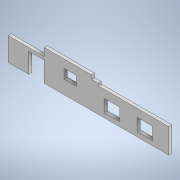
# Autodesk Inventor part: eastSideofHouseFacingPool
Saved by Autodesk Inventor 2020.1 (Build 241239000, 239)
## iProperties
Created: 2019-08-10
Part Number: eastSideofHouseFacingPool
Material: Generic
Document SubType Name: Modeling
Designer: steele
Density: 1 g/cm^3
Appearance: Default
Mass: 1.01363e+07 g
Surface Area: 838837 cm^2
Volume: 1.01363e+07 cm^3
Author: steele
Autodesk Inventor part; units mm, degrees
ref_plane "YZ Plane" through (0, 0, 0) normal (1, 0, 0) x (0, 1, 0)
ref_plane "XZ Plane" through (0, 0, 0) normal (0, 1, 0) x (-1, 0, 0)
ref_plane "XY Plane" through (0, 0, 0) normal (0, 0, 1) x (1, 0, 0)
sketch "Sketch2" plane through (0, 0, 0) normal (0, 0, 1) x (1, 0, 0)
  line L0 (0, 0) -> (2032, 0)
  line L1 (2032, 0) -> (2032, 1981.2)
  line L2 (2032, 2286) -> (0, 2286)
  line L3 (0, 2286) -> (0, 0)
  line L4 (2032, 2286) -> (3556, 2286)
  line L5 (3556, 1981.2) -> (2032, 1981.2)
  line L6 (3556, 1981.2) -> (3556, 0) construction
  line L7 (3556, 0) -> (8204.2, 0)
  line L8 (8229.6, 2667) -> (8229.6, 3048)
  line L9 (8229.6, 3048) -> (3556, 3048)
  line L10 (8204.2, 0) -> (8864.6, 0)
  line L11 (8890, 2438.4) -> (8890, 2667)
  line L12 (8890, 2667) -> (8229.6, 2667)
  line L13 (8864.6, 0) -> (15849.6, 0)
  line L14 (15849.6, 0) -> (15849.6, 2438.4)
  line L15 (15849.6, 2438.4) -> (8890, 2438.4)
  line L16 (9492.6899, 457.2) -> (11016.6899, 457.2)
  line L17 (11016.6899, 457.2) -> (11016.6899, 1676.4)
  line L18 (11016.6899, 1676.4) -> (9492.6899, 1676.4)
  line L19 (9492.6899, 1676.4) -> (9492.6899, 457.2)
  line L20 (9492.6899, 457.2) -> (11016.6899, 1676.4) construction
  line L21 (11016.6899, 457.2) -> (9492.6899, 1676.4) construction
  line L22 (12725.2645, 457.2) -> (14249.2645, 457.2)
  line L23 (14249.2645, 457.2) -> (14249.2645, 1676.4)
  line L24 (14249.2645, 1676.4) -> (12725.2645, 1676.4)
  line L25 (12725.2645, 1676.4) -> (12725.2645, 457.2)
  line L26 (12725.2645, 457.2) -> (14249.2645, 1676.4) construction
  line L27 (14249.2645, 457.2) -> (12725.2645, 1676.4) construction
  line L28 (5522.7071, 1352.1351) -> (6741.9071, 1352.1351)
  line L29 (6741.9071, 1352.1351) -> (6741.9071, 2266.5351)
  line L30 (6741.9071, 2266.5351) -> (5522.7071, 2266.5351)
  line L31 (5522.7071, 1352.1351) -> (6741.9071, 2266.5351) construction
  line L32 (6741.9071, 1352.1351) -> (5522.7071, 2266.5351) construction
  line L33 (5522.7071, 2266.5351) -> (5522.7071, 1981.2)
  line L34 (5522.7071, 1676.4) -> (5522.7071, 1352.1351)
  line L35 (3556, 3048) -> (3556, 2286)
  line L36 (3556, 1981.2) -> (3556, 0)
  line L37 (5522.7071, 2266.5351) -> (5522.7071, 1352.1351)
  point P0 (10254.6899, 1066.8)
  point P1 (13487.2645, 1066.8)
  point P2 (6132.3071, 1809.3351)
  dimension "d25" = 2286
  dimension "d26" = 1524
  dimension "d28" = 4673.6
  dimension "d34" = 6959.6
  dimension "d35" = 2438.4
  dimension "d36" = 1524
  dimension "d38" = 1219.2
  dimension "d39" = 1524
  dimension "d40" = 1219.2
  dimension "d41" = 1219.2
  dimension "d42" = 914.4
  dimension "d43" = 660.4
  dimension "d44" = 2667
  dimension "d45" = 3048
  dimension "d46" = 304.8
  dimension "d51" = 3556
  dimension "d52" = 2032
  dimension "d53" = 12293.6
  constraints: 76 end point, 15 parallel, 8 horizontal, 7 perpendicular, 6 midpoint, 2 point on line, 2 vertical, 1 collinear
  measures "d25" distance of L2.start L0.end
  measures "d26" distance of L1.end L5.start
  measures "d28" distance of L9.end L8.end
  measures "d34" distance of L11.start L14.end
  measures "d35" distance of L14.end L13.end
  measures "d36" distance of L16.start L16.end
  measures "d38" distance of L16.end L17.end
  measures "d39" distance of L22.start L22.end
  measures "d40" distance of L23.end L22.end
  measures "d41" distance of L28.start L28.end
  measures "d42" distance of L29.end L28.end
  measures "d43" distance of L11.end L8.start
  measures "d44" distance from line of L10.end L12
  measures "d45" distance between parallel lines of L7 L9
  measures "d46" distance between parallel lines of L4 L5
  measures "d51" distance between parallel lines of L35 L3
  measures "d52" distance between parallel lines of L3 L1
  measures "d53" distance of L6.end L13.end
extrude "Extrusion2" add sketch "Sketch2" against normal blind 304.8
body "Solid2"
